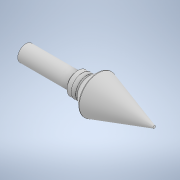
# Autodesk Inventor part: Weapon-Projectile-Barrel
Saved by Autodesk Inventor 2020 (Build 240168000, 168)
## iProperties
Created: 2019-11-08
Part Number: Weapon-Projectile-Barrel
Material: Generic
Document SubType Name: Modeling
Designer: vifly_01
Density: 1 g/cm^3
Appearance: Default
Author: vifly_01
Autodesk Inventor part; units mm, degrees
ref_plane "YZ Plane" through (0, 0, 0) normal (1, 0, 0) x (0, 1, 0)
ref_plane "XZ Plane" through (0, 0, 0) normal (0, 1, 0) x (-1, 0, 0)
ref_plane "XY Plane" through (0, 0, 0) normal (0, 0, 1) x (1, 0, 0)
sketch "Sketch1" plane through (0, 0, 0) normal (0, 0, 1) x (1, 0, 0)
  circle A0 centre (0, 0) radius 6.5
  dimension "d0" = 13
  constraints: 1 centre point, 1 coincident
  measures "d0" diameter of A0
extrude "Extrusion1" add sketch "Sketch1" along normal blind 40
sketch "Sketch2" plane through (0, 0, 40) normal (0, 0, 1) x (1, 0, 0)
  circle A0 centre (0, 0) radius 6.5
  circle A1 centre (0, 0) radius 6.5 projected
  dimension "d29" = 0
  constraints: 1 centre point, 1 coincident
  measures "d29" radial gap between concentric circles of A1 A0
extrude "Extrusion2" add sketch "Sketch2" along normal blind 2 draft 50
sketch "Sketch3" plane through (0, 0, 42) normal (0, 0, 1) x (1, 0, 0)
  circle A0 centre (0, 0) radius 8.8835
  circle A1 centre (0, 0) radius 8.8835 projected
  dimension "d30" = 0
  constraints: 1 centre point, 1 coincident
  measures "d30" radial gap between concentric circles of A1 A0
extrude "Extrusion3" add sketch "Sketch3" along normal blind 3.5
sketch "Sketch4" plane through (0, 0, 45.5) normal (0, 0, 1) x (1, 0, 0)
  circle A0 centre (0, 0) radius 8.9835
  circle A1 centre (0, 0) radius 8.8835 projected
  dimension "d23" = 0.1
  constraints: 1 centre point, 1 coincident
  measures "d23" radial gap between concentric circles of A0 A1
extrude "Extrusion4" add sketch "Sketch4" along normal blind 3.5 contours A0 | A1
sketch "Sketch5" plane through (0, 0, 49) normal (0, 0, 1) x (1, 0, 0)
  circle A0 centre (0, 0) radius 8.8835
  circle A1 centre (0, 0) radius 8.9835 projected
  circle A2 centre (0, 0) radius 8.8835 projected
  dimension "d25" = 0
  constraints: 1 centre point, 1 coincident
  measures "d25" radial gap between concentric circles of A0 A2
extrude "Extrusion5" add sketch "Sketch5" along normal blind 1.25 contours A0
sketch "Sketch6" plane through (0, 0, 50.25) normal (0, 0, 1) x (1, 0, 0)
  circle A0 centre (0, 0) radius 8.8835
  circle A1 centre (0, 0) radius 8.8835 projected
  dimension "d26" = 0
  constraints: 1 centre point, 1 coincident
  measures "d26" radial gap between concentric circles of A0 A1
extrude "Extrusion6" add sketch "Sketch6" along normal blind 7.5 draft 40
sketch "Sketch7" plane through (0, 0, 57.75) normal (0, 0, 1) x (1, 0, 0)
  circle A0 centre (0, 0) radius 15.1768
  circle A1 centre (0, 0) radius 15.1768 projected
  dimension "d27" = 0
  constraints: 1 centre point, 1 coincident
  measures "d27" radial gap between concentric circles of A0 A1
extrude "Extrusion7" add sketch "Sketch7" along normal blind 0.5
sketch "Sketch8" plane through (0, 0, 58.25) normal (0, 0, 1) x (1, 0, 0)
  circle A0 centre (0, 0) radius 15.1768
  circle A1 centre (0, 0) radius 15.1768 projected
  dimension "d31" = 0
  constraints: 1 centre point, 1 coincident
  measures "d31" radial gap between concentric circles of A1 A0
extrude "Extrusion8" add sketch "Sketch8" along normal blind 45 draft -17.5
body "Solid1"
